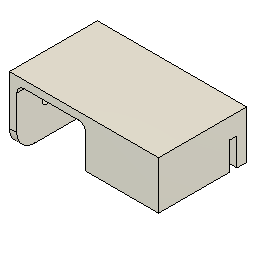
Servo Pot Holder (Autodesk Fusion 360 design; units mm, degrees)
Autodesk Fusion 360 part; units mm, degrees
note: some values were not read from the file. Chosen so that the rebuilt part matches the saved one: a direction; which pieces of a blend or face edit are solid. Set by a fixed rule: which sketch regions a step uses.
sketch "Sketch1" plane through (0, 0, 0) normal (0, 1, 0) x (1, 0, 0)
  line L0 (0, 0) -> (41.275, 0)
  line L1 (41.275, 0) -> (41.275, -30.7975)
  line L2 (41.275, -30.7975) -> (0, -30.7975)
  line L3 (0, -30.7975) -> (0, 0)
  line L4 (5.334, -2.54) -> (38.1, -2.54)
  line L5 (38.1, -2.54) -> (38.1, -30.7975)
  line L6 (38.1, -30.7975) -> (5.334, -30.7975)
  line L7 (5.334, -30.7975) -> (5.334, -2.54)
  dimension "d1" = 41.275
  dimension "d2" = 30.7975
  dimension "d3" = 5.334
  dimension "d4" = 3.175
  dimension "d5" = 2.54
  measures "d3" distance of L3 L7
  measures "d4" distance of L1 L5
  measures "d5" distance of L0 L4
extrude "Extrude1" add sketch "Sketch1" along normal blind 17.145 contours L0 L1 L2 L3 L4 L5 L7 makes body 1
sketch "Sketch2" plane through (0, 0, 0) normal (-1, 0, 0) x (0, 0, 1)
  line L0 (0, 0) -> (30.7975, 0)
  line L1 (30.7975, 0) -> (30.7975, 17.145)
  line L2 (30.7975, 17.145) -> (0, 17.145)
  line L3 (0, 17.145) -> (0, 0)
  circle A0 centre (22.225, 8.5725) radius 8.5725
extrude "Extrude2" cut sketch "Sketch2" against normal through all contours L0 L1 A0 | L1 L2 A0 bodies 1
sketch "Sketch3" plane through (38.1, 0, 0) normal (-1, 0, 0) x (0, 0, 1)
  arc A0 (22.225, 0) -> (22.225, 17.145) centre (22.225, 8.5725) ccw
  line L0 (22.225, 17.145) -> (2.54, 17.145)
  line L1 (2.54, 17.145) -> (2.54, 0)
  line L2 (2.54, 0) -> (22.225, 0)
  circle A1 centre (22.225, 8.5725) radius 6.0325
  dimension "d9" = 12.065
  measures "d9" diameter of A1
extrude "Extrude3" cut sketch "Sketch3" against normal blind 2.54 contours A1 bodies 1
sketch "Sketch4" plane through (0, 0, 0) normal (-1, 0, 0) x (0, 0, 1)
  arc A0 (22.225, 0) -> (22.225, 17.145) centre (22.225, 8.5725) ccw
  line L0 (22.225, 17.145) -> (0, 17.145)
  line L1 (0, 17.145) -> (0, 0)
  line L2 (0, 0) -> (22.225, 0)
  circle A1 centre (22.225, 8.5725) radius 3.556 construction
  line L3 (25.781, 8.5725) -> (5.969, 8.5725) construction
  line L4 (20.1084, 11.43) -> (20.1084, 5.715) construction
  circle A2 centre (5.969, 8.5725) radius 2.032 construction
  line L5 (20.1084, 11.43) -> (5.8511, 10.6011)
  line L6 (20.1084, 5.715) -> (5.8511, 6.5439)
  circle A3 centre (5.969, 8.5725) radius 0.5715
  circle A4 centre (8.255, 8.5725) radius 0.5715
  circle A5 centre (10.541, 8.5725) radius 0.5715
  circle A6 centre (12.827, 8.5725) radius 0.5715
  circle A7 centre (15.113, 8.5725) radius 0.5715
  circle A8 centre (17.399, 8.5725) radius 0.5715
  arc A9 (5.8511, 10.6011) -> (5.8511, 6.5439) centre (5.969, 8.5725) ccw
  arc A10 (20.1084, 5.715) -> (20.1084, 11.43) centre (22.225, 8.5725) ccw
  arc A11 (5.8216, 11.1082) -> (5.8216, 6.0368) centre (5.969, 8.5725) ccw
  line L7 (19.9332, 5.2163) -> (5.8216, 6.0368)
  arc A12 (19.9332, 5.2163) -> (19.9332, 11.9287) centre (22.225, 8.5725) ccw
  line L8 (19.9332, 11.9287) -> (5.8216, 11.1082)
  circle A13 centre (22.225, 8.5725) radius 4.064
  dimension "d13" = 7.112
  dimension "d14" = 19.812
  dimension "d15" = 5.715
  dimension "d16" = 4.064
  dimension "d17" = 1.143
  dimension "d20" = 11.43
  dimension "d21" = 0
  dimension "d22" = 0.508
  measures "d13" diameter of A1
  measures "d16" diameter of A2
  measures "d17" diameter of A3
extrude "Extrude4" cut sketch "Sketch4" against normal blind 3.81 contours L5 L6 A10 A13 | L5 L6 A10 A12 A13 | L5 L6 A9 A13 | L5 L6 A9 A11 L7 L8 A13 | A3 | A4 | A5 | A6 | A7 | A8 bodies 1
fillet "Fillet2" radius 6.35 2 edges at (5.334, 8.5725, 2.54) (38.1, 8.5725, 2.54) on bodies 1
extrude "Extrude5" cut sketch "Sketch4" against normal blind 12.7 contours L5 L6 A10 A13 | L5 L6 A10 A12 A13 | A3 | A4 | A5 | A6 | A7 | A8 bodies 1
sketch "Sketch8" plane through (0, 17.145, 0) normal (0, 1, 0) x (-1, 0, 0)
  line L0 (-38.1, 22.225) -> (-41.275, 22.225)
  line L1 (-41.275, 22.225) -> (-41.275, 0)
  line L2 (-41.275, 0) -> (0, 0)
  line L3 (0, 0) -> (0, 22.225)
  line L4 (0, 22.225) -> (-5.334, 22.225)
  line L5 (-5.334, 22.225) -> (-5.334, 8.89)
  arc A0 (-11.684, 2.54) -> (-5.334, 8.89) centre (-11.684, 8.89) ccw
  line L6 (-11.684, 2.54) -> (-31.75, 2.54)
  arc A1 (-38.1, 8.89) -> (-31.75, 2.54) centre (-31.75, 8.89) ccw
  line L7 (-38.1, 8.89) -> (-38.1, 22.225)
  line L8 (-37.592, 2.54) -> (-6.604, 2.54)
  line L9 (-6.604, 2.54) -> (-6.604, -34.925)
  line L10 (-6.604, -34.925) -> (-37.592, -34.925)
  line L11 (-37.592, -34.925) -> (-37.592, 2.54)
  dimension "d48" = 30.988
  dimension "d49" = 37.465
  dimension "d50" = 6.604
  measures "d49" distance of L2.end
  measures "d50" distance of L3 L9
extrude "Extrude8" add sketch "Sketch8" against normal blind 17.145 contours L2 L9 L10 L11 bodies 1
sketch "Sketch9" plane through (37.592, 0, 0) normal (1, 0, 0) x (0, 0, -1)
  line L0 (34.925, 17.145) -> (0, 17.145)
  line L1 (0, 17.145) -> (0, 0)
  line L2 (0, 0) -> (34.925, 0)
  line L3 (34.925, 0) -> (34.925, 17.145)
  line L4 (0, 8.5725) -> (34.925, 8.5725) construction
  circle A0 centre (21.2725, 8.5725) radius 14.9225
  dimension "d53" = 29.845
  dimension "d55" = 28.575
  measures "d53" diameter of A0
  measures "d55" distance of L3
extrude "Extrude9" add sketch "Sketch9" along normal blind -37.592 and the other way blind -3.683 contours L0 L1 L2 A0 bodies 1
sketch "Sketch11" plane through (5.334, 0, 0) normal (1, 0, 0) x (0, 0, -1)
  circle A0 centre (-15.113, 8.5725) radius 0.5715
  circle A1 centre (-12.827, 8.5725) radius 0.5715
  circle A2 centre (-17.399, 8.5725) radius 0.5715
  circle A3 centre (-10.541, 8.5725) radius 0.5715
  circle A4 centre (-22.225, 8.5725) radius 4.064
  line L0 (-8.89, 0) -> (-8.89, 17.145)
  line L1 (-8.89, 17.145) -> (-22.225, 17.145)
  arc A5 (-22.225, 17.145) -> (-22.225, 0) centre (-22.225, 8.5725) ccw
  line L2 (-22.225, 0) -> (-8.89, 0)
  line L3 (-5.8216, 11.1082) -> (-19.9332, 11.9287)
  arc A6 (-19.9332, 11.9287) -> (-19.9332, 5.2163) centre (-22.225, 8.5725) ccw
  line L4 (-19.9332, 5.2163) -> (-5.8216, 6.0368)
  arc A7 (-5.8216, 6.0368) -> (-5.8216, 11.1082) centre (-5.969, 8.5725) ccw
  line L5 (9.058, 0) -> (-22.225, 0)
  arc A8 (-22.225, 17.145) -> (-22.225, 0) centre (-22.225, 8.5725) ccw
  line L6 (-22.225, 17.145) -> (9.058, 17.145)
  line L7 (-19.9332, 5.2163) -> (-22.225, 0)
  line L8 (-19.9332, 11.9287) -> (-22.225, 17.145)
  arc A9 (9.058, 17.145) -> (9.058, 0) centre (21.2725, 8.5725) ccw
extrude "Extrude10" cut sketch "Sketch11" against normal blind 2.54 contours A4 A5 A6 A8 L7 L8 bodies 1
chamfer "Chamfer4" distance 2.54 distance2 6.35 2 edges at (2.794, 14.5368, 21.0791) (2.794, 2.6082, 21.0791) measured on face at (3.9793, 15.4062, 21.4611) measured on face at (3.9793, 1.7388, 21.4611) on bodies 1
sketch "Sketch13" plane through (0, 0, 0) normal (0, -1, 0) x (1, 0, 0)
  line L0 (5.334, 22.225) -> (0, 22.225)
  line L1 (0, 22.225) -> (0, -9.058)
  line L2 (6.604, -9.058) -> (6.604, -34.925)
  line L3 (6.604, -34.925) -> (37.592, -34.925)
  line L4 (37.592, -34.925) -> (37.592, -9.058)
  line L5 (41.275, -9.058) -> (41.275, 22.225)
  line L6 (41.275, 22.225) -> (38.1, 22.225)
  line L7 (37.592, -34.925) -> (6.604, -34.925)
  line L8 (6.604, -34.925) -> (6.604, 2.54)
  line L9 (6.604, 2.54) -> (37.592, 2.54)
  line L10 (37.592, 2.54) -> (37.592, -34.925)
  line L11 (0, -9.058) -> (6.604, -9.058)
  line L12 (37.592, -9.058) -> (41.275, -9.058)
  line L13 (38.1, 22.225) -> (38.1, 8.89)
  arc A0 (31.75, 2.54) -> (38.1, 8.89) centre (31.75, 8.89) ccw
  arc A1 (5.334, 8.89) -> (11.684, 2.54) centre (11.684, 8.89) ccw
  line L14 (5.334, 8.89) -> (5.334, 22.225)
  line L15 (11.684, 2.54) -> (31.75, 2.54)
extrude "Extrude12" cut sketch "Sketch13" against normal blind 3.048 contours L2 L3 L4 L7 L8 L9 L10 L15 bodies 1
sketch "Sketch14" plane through (0, 3.048, 0) normal (0, -1, 0) x (1, 0, 0)
  line L0 (11.684, 2.54) -> (6.604, 2.54)
  line L1 (6.604, 2.54) -> (6.604, -7.4103)
  line L2 (6.604, -7.4103) -> (6.604, -34.925)
  line L3 (6.604, -34.925) -> (37.592, -34.925)
  line L4 (37.592, -34.925) -> (37.592, -7.4103)
  line L5 (37.592, -7.4103) -> (37.592, 2.54)
  line L6 (35.052, -30.7975) -> (25.527, -30.7975)
  line L7 (25.527, -30.7975) -> (25.527, -1.5875)
  line L8 (25.527, -1.5875) -> (35.052, -1.5875)
  line L9 (35.052, -1.5875) -> (35.052, -30.7975)
  line L10 (22.098, -34.925) -> (22.098, 2.54) construction
  line L11 (9.144, -16.1925) -> (35.052, -16.1925) construction
  line L12 (22.352, -28.0035) -> (15.3035, -28.0035)
  line L13 (15.3035, -28.0035) -> (15.3035, -4.3815)
  line L14 (15.3035, -4.3815) -> (22.352, -4.3815)
  line L15 (22.352, -4.3815) -> (22.352, -28.0035)
  line L16 (15.3035, -32.9565) -> (12.6365, -32.9565)
  line L17 (12.6365, -32.9565) -> (12.6365, 0.5715)
  line L18 (12.6365, 0.5715) -> (15.3035, 0.5715)
  line L19 (15.3035, 0.5715) -> (15.3035, -32.9565)
  line L20 (25.527, -1.5875) -> (22.352, -4.3815)
  line L21 (25.527, -30.7975) -> (22.352, -28.0035)
  line L22 (13.97, -32.9565) -> (13.97, 0.5715) construction
  line L23 (15.3035, -28.0035) -> (12.6365, -28.0035) construction
  line L24 (15.3035, -4.3815) -> (12.6365, -4.3815) construction
  line L25 (12.6365, -28.0035) -> (6.604, -28.0035)
  line L26 (6.604, -28.0035) -> (6.604, -12.2555)
  line L27 (6.604, -12.2555) -> (12.6365, -12.2555) construction
  line L28 (12.6365, -12.2555) -> (12.6365, -28.0035)
  line L29 (12.6365, -4.3815) -> (11.049, -4.3815)
  line L30 (6.604, -12.2555) -> (10.414, -12.2555)
  line L31 (11.049, -4.3815) -> (10.414, -12.2555)
  circle A0 centre (22.098, -30.48) radius 1.143
  circle A1 centre (22.098, -1.905) radius 1.143
  line L32 (37.592, 2.54) -> (31.75, 2.54)
  line L33 (11.684, 2.54) -> (31.75, 2.54)
  line L34 (12.6365, -4.3815) -> (6.604, -4.3815)
  line L35 (12.6365, -28.0035) -> (11.049, -28.0035)
  line L36 (6.604, -20.1295) -> (10.414, -20.1295)
  line L37 (10.414, -20.1295) -> (11.049, -28.0035)
  dimension "d73" = 2.54
  dimension "d74" = 29.21
  dimension "d75" = 9.525
  dimension "d76" = 12.7
  dimension "d78" = 2.794
  dimension "d79" = 4.953
  dimension "d80" = 7.366
  dimension "d81" = 2.667
  dimension "d82" = 15.748
  dimension "d83" = 1.5875
  dimension "d84" = 3.81
  dimension "d85" = 2.286
  dimension "d86" = 2.286
  dimension "d87" = 4.445
  dimension "d88" = 4.445
  dimension "d122" = 2.794
  dimension "d130" = 1.5875
  dimension "d131" = 3.81
  dimension "d132" = 15.748
  measures "d73" distance of L4 L9
  measures "d74" distance of origin
  measures "d76" distance of L9 origin
  measures "d80" distance of L2
  measures "d85" diameter of A0
  measures "d86" diameter of A1
  measures "d132" distance of L36
extrude "Extrude13" cut sketch "Sketch14" against normal blind 11.557 contours L2 L17 L25 L26 L28 L29 L30 L31 L34 L35 L36 L37 | L13 L16 L17 L18 L19 L28 | L2 L25 L26 L36 L37 | L12 L13 L14 L15 L19 | L7 L15 L20 L21 | L6 L7 L8 L9 | A0 | A1 bodies 1
sketch "Sketch21" plane through (37.592, 0, 0) normal (1, 0, 0) x (0, 0, -1)
  line L0 (7.4103, 3.048) -> (34.925, 3.048) construction
  circle A0 centre (21.5011, 8.5725) radius 3.81
  line L1 (24.3409, 6.0325) -> (18.6613, 6.0325)
  line L2 (18.6613, 6.0325) -> (18.6613, 11.1125)
  line L3 (18.6613, 11.1125) -> (24.3409, 11.1125)
  line L4 (24.3409, 11.1125) -> (24.3409, 6.0325)
  line L5 (1.5875, 3.048) -> (30.7975, 3.048)
  line L6 (16.1925, 3.048) -> (16.1925, 17.145) construction
  line L7 (34.925, 3.048) -> (34.925, 17.145)
  line L8 (34.925, 17.145) -> (9.058, 17.145)
  arc A1 (9.058, 17.145) -> (7.4103, 3.048) centre (21.2725, 8.5725) ccw
  dimension "d115" = 7.62
  dimension "d116" = 5.08
  dimension "d118" = 5.3086
  dimension "d123" = 8.5725
  measures "d115" diameter of A0
  measures "d116" distance of L1 L3
  measures "d118" distance of L6
extrude "Extrude17" add sketch "Sketch21" along normal blind 2.794 contours A0 L4 | L1 L2 L3 L4 | A0 L2 bodies 1
sketch "Sketch22" plane through (0, 0, 0) normal (0, -1, 0) x (1, 0, 0)
  line L0 (37.592, 2.54) -> (37.592, -9.058)
  line L1 (37.592, -9.058) -> (41.275, -9.058)
  line L2 (41.275, -9.058) -> (41.275, 22.225)
  line L3 (41.275, 22.225) -> (38.1, 22.225)
  line L4 (31.75, 2.54) -> (37.592, 2.54)
  line L5 (37.592, -34.925) -> (6.604, -34.925)
  line L6 (6.604, -34.925) -> (6.604, 2.54)
  line L7 (6.604, 2.54) -> (37.592, 2.54)
  line L8 (37.592, 2.54) -> (37.592, -34.925)
  line L9 (41.275, -9.058) -> (0, -9.058)
  line L10 (0, -9.058) -> (0, 35.392)
  line L11 (0, 35.392) -> (41.275, 35.392)
  line L12 (41.275, 35.392) -> (41.275, -9.058)
  line L13 (0, -9.058) -> (0, 22.225)
  line L14 (38.1, 22.225) -> (38.1, 8.89)
  arc A0 (31.75, 2.54) -> (38.1, 8.89) centre (31.75, 8.89) ccw
  dimension "d125" = 44.45
  measures "d125" distance of origin
extrude "Extrude18" cut sketch "Sketch22" against normal through all contours L0 L1 L2 L3 L4 L7 L8 L9 L12 L14 A0 | L3 L6 L7 L9 L10 L11 L12 L13 L14 A0 bodies 1
sketch "Sketch24" plane through (0, 3.048, 0) normal (0, -1, 0) x (1, 0, 0)
  line L0 (12.6365, -28.0035) -> (6.604, -28.0035)
  line L1 (6.604, -28.0035) -> (6.604, -34.925)
  line L2 (6.604, -34.925) -> (37.592, -34.925)
  line L3 (37.592, -34.925) -> (37.592, 2.54)
  line L4 (37.592, 2.54) -> (6.604, 2.54)
  line L5 (6.604, 2.54) -> (6.604, -12.2555)
  line L6 (6.604, -12.2555) -> (10.414, -12.2555)
  line L7 (10.414, -12.2555) -> (11.049, -4.3815)
  line L8 (11.049, -4.3815) -> (12.6365, -4.3815)
  line L9 (12.6365, -4.3815) -> (12.6365, 0.5715)
  line L10 (12.6365, 0.5715) -> (15.3035, 0.5715)
  line L11 (15.3035, 0.5715) -> (15.3035, -4.3815)
  line L12 (15.3035, -4.3815) -> (22.352, -4.3815)
  line L13 (22.352, -4.3815) -> (25.527, -1.5875)
  line L14 (25.527, -1.5875) -> (35.052, -1.5875)
  line L15 (35.052, -1.5875) -> (35.052, -30.7975)
  line L16 (35.052, -30.7975) -> (25.527, -30.7975)
  line L17 (25.527, -30.7975) -> (22.352, -28.0035)
  line L18 (22.352, -28.0035) -> (15.3035, -28.0035)
  line L19 (15.3035, -28.0035) -> (15.3035, -32.9565)
  line L20 (15.3035, -32.9565) -> (12.6365, -32.9565)
  line L21 (12.6365, -32.9565) -> (12.6365, -28.0035)
  circle A0 centre (22.098, -30.48) radius 1.143
  circle A1 centre (22.098, -1.905) radius 1.143
  line L22 (35.052, -1.5875) -> (35.687, -1.5875)
  line L23 (35.687, -1.5875) -> (35.687, -30.7975)
  line L24 (35.687, -30.7975) -> (35.052, -30.7975)
  line L25 (35.052, -30.7975) -> (35.052, -1.5875)
  dimension "d133" = 0.635
extrude "Extrude20" cut sketch "Sketch24" against normal blind 11.557 contours L15 L22 L23 L24 L25 bodies 1
extrude "Extrude21" cut 1 faces at (31.242, 14.605, -20.1295) along direction (0, 1, 0) blind 0.254 on bodies 1 bodies 1
sketch "Sketch26" plane through (35.687, 0, 0) normal (-1, 0, 0) x (0, 0, 1)
  line L0 (-30.7975, 3.048) -> (-1.5875, 3.048)
  line L1 (-1.5875, 3.048) -> (-1.5875, 14.859)
  line L2 (-1.5875, 14.859) -> (-30.7975, 14.859)
  line L3 (-30.7975, 14.859) -> (-30.7975, 3.048)
  line L4 (-30.7975, 3.048) -> (-27.7975, 3.048)
  line L5 (-27.7975, 3.048) -> (-27.7975, 14.859)
  line L6 (-27.7975, 14.859) -> (-30.7975, 14.859)
  line L7 (-30.7975, 14.859) -> (-30.7975, 3.048)
  dimension "d140" = 3
extrude "Extrude23" cut sketch "Sketch26" against normal blind 1.905 contours L0 L2 L3 L4 L5 L6 L7 bodies 1
move_face "OffsetFaces1" offset 6.35 1 faces at (27.2627, 17.145, -22.4367) on bodies 1
sketch "Sketch27" plane through (0, 23.495, 0) normal (0, 1, 0) x (-1, 0, 0)
  line L0 (-37.592, 2.54) -> (-37.592, -34.925)
  line L1 (-37.592, -34.925) -> (-6.604, -34.925)
  line L2 (-6.604, -34.925) -> (-6.604, 2.54)
  line L3 (-6.604, 2.54) -> (-37.592, 2.54)
  line L4 (-37.592, -34.925) -> (25.908, -34.925)
  line L5 (25.908, -34.925) -> (25.908, 2.54)
  line L6 (25.908, 2.54) -> (-37.592, 2.54)
  line L7 (-37.592, 2.54) -> (-37.592, -34.925)
  dimension "d144" = 63.5
extrude "Extrude24" add sketch "Sketch27" against normal blind 3.175 contours L2 L4 L5 L6 bodies 1
sketch "Sketch28" plane through (0, 20.32, 0) normal (0, -1, 0) x (1, 0, 0)
  line L0 (-25.908, -34.925) -> (6.604, -34.925)
  line L1 (6.604, -34.925) -> (6.604, 2.54)
  line L2 (6.604, 2.54) -> (-25.908, 2.54)
  line L3 (-25.908, 2.54) -> (-25.908, -34.925)
  line L4 (-25.908, 2.54) -> (-22.733, 2.54)
  line L5 (-22.733, 2.54) -> (-22.733, -34.925)
  line L6 (-22.733, -34.925) -> (-25.908, -34.925)
  line L7 (-25.908, -34.925) -> (-25.908, 2.54)
  dimension "d147" = 3.175
extrude "Extrude25" add sketch "Sketch28" along normal blind 25.4 contours L0 L2 L3 L4 L5 L6 L7 bodies 1
sketch "Sketch29" plane through (-25.908, 0, 0) normal (-1, 0, 0) x (0, 0, 1)
  line L0 (2.54, 23.495) -> (-34.925, 23.495)
  line L1 (-34.925, 23.495) -> (-34.925, -5.08)
  line L2 (-34.925, -5.08) -> (2.54, -5.08)
  line L3 (2.54, -5.08) -> (2.54, 23.495)
  arc A0 (-18.6613, 6.0325) -> (-18.6613, 11.1125) centre (-21.5011, 8.5725) ccw
  arc A1 (-24.3409, 11.1125) -> (-24.3409, 6.0325) centre (-21.5011, 8.5725) ccw
  circle A2 centre (-21.5011, 8.5725) radius 3.9688
  circle A3 centre (-10.2299, 8.5725) radius 1.905
  line L4 (-21.5011, 8.5725) -> (-10.2299, 8.5725) construction
  line L5 (-21.5011, 8.5725) -> (-25.4699, 8.5725) construction
  dimension "d150" = 7.9375
  dimension "d153" = 3.81
  dimension "d154" = 15.24
  measures "d150" diameter of A2
  measures "d153" diameter of A3
extrude "Extrude26" cut sketch "Sketch29" against normal blind 3.175 contours A2 | A3 bodies 1
fillet "Fillet11" radius 7.62 2 edges at (-24.3205, -5.08, 2.54) (-24.3205, -5.08, -34.925) on bodies 1
extrude "Extrude27" add 2 faces at (21.4964, 14.605, -30.8127) (21.9588, 14.605, -2.2597) along direction (0, -1, 0) blind 11.557 on bodies 1 bodies 1
sketch "Sketch1 (2)" plane through (0, 0, 0) normal (0, 1, 0) x (1, 0, 0) in component "Shaft Adapter"
  circle A0 centre (0, 0) radius 5.08
  circle A1 centre (0, 0) radius 1.27
  circle A2 centre (0, 0) radius 2.3813
  dimension "d158" = 2.54
  dimension "d159" = 10.16
  dimension "d160" = 4.7625
  measures "d158" diameter of A1
  measures "d159" diameter of A0
  measures "d160" diameter of A2
extrude "Extrude1'" add sketch "Sketch1 (2)" against normal blind 3.175 separate body contours A0 makes body 2 in component "Shaft Adapter"
sketch "Sketch2 (2)" plane through (0, -3.175, 0) normal (0, -1, 0) x (1, 0, 0) in component "Shaft Adapter"
  circle A0 centre (0, 0) radius 2.3813
  circle A1 centre (0, 0) radius 5.08
  circle A2 centre (0, 0) radius 1.27
extrude "Extrude2'" add sketch "Sketch2 (2)" along normal blind 1.5 contours A0 | A1 bodies 2 in component "Shaft Adapter"
sketch "Sketch3 (2)" plane through (0, -4.675, 0) normal (0, -1, 0) x (1, 0, 0) in component "Shaft Adapter"
  circle A0 centre (0, 0) radius 1.27
  circle A1 centre (0, 0) radius 5.08
  circle A2 centre (0, 0) radius 3.175
  line L0 (-2.5981, 1.825) -> (2.5981, 1.825)
  line L1 (0, 0) -> (0, -3.175)
  circle A3 centre (0, 0) radius 1.9685
  dimension "d165" = 6.35
  dimension "d166" = 5
  dimension "d167" = 3.937
  measures "d165" diameter of A2
  measures "d166" distance of L0
  measures "d167" diameter of A3
extrude "Extrude3'" add sketch "Sketch3 (2)" along normal blind 9.525 contours A1 | A2 L0 A3 bodies 2 in component "Shaft Adapter"
extrude "Extrude28" cut 1 faces at (40.386, 9.4192, -20.5545) along direction (-1, 0, 0) blind 2.794 on bodies 1 bodies 1
fillet "Fillet12" radius 3.175 2 edges at (6.604, 20.32, -16.1925) (-22.733, 20.32, -16.1925) on bodies 1
sketch "Sketch4 (2)" plane through (0, -14.2, 0) normal (0, -1, 0) x (1, 0, 0) in component "Shaft Adapter"
  arc A0 (-2.5981, 1.825) -> (2.5981, 1.825) centre (0, 0) ccw
  line L0 (-2.5981, 1.825) -> (-0.7378, 1.825)
  arc A1 (0.7378, 1.825) -> (-0.7378, 1.825) centre (0, 0) ccw
  line L1 (0.7378, 1.825) -> (2.5981, 1.825)
  circle A2 centre (0, 0) radius 5.08
  line L2 (2.9329, 5.08) -> (-2.9329, 5.08)
  line L3 (-2.9329, 5.08) -> (-5.8659, 0)
  line L4 (-5.8659, 0) -> (-2.9329, -5.08)
  line L5 (-2.9329, -5.08) -> (2.9329, -5.08)
  line L6 (2.9329, -5.08) -> (5.8659, 0)
  line L7 (5.8659, 0) -> (2.9329, 5.08)
  circle A3 centre (0, 0) radius 5.08
extrude "Extrude4'" add sketch "Sketch4 (2)" against normal blind 14.2 contours A2 L6 L7 A3 | A2 L2 L7 A3 | A2 L5 L6 A3 | A2 L2 L3 A3 | A2 L4 L5 A3 | A2 L3 L4 A3 bodies 2 in component "Shaft Adapter"
component "Shaft Adapter" placed x (0, 1, 0) y (1, 0, 0) z (0, 0, -1) at (4.167, 8.5725, -21.5011)
equation "d48 = 1.213 in + 0.007 in"
equation "d79 = 0.175 in + 0.02 in"
